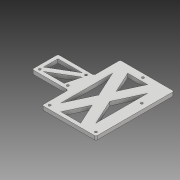
# Autodesk Inventor part: soporte_nuc_up
Saved by Autodesk Inventor 2018 (Build 220112000, 112)
## iProperties
Created: 2019-01-10
Part Number: soporte_nuc_up
Material: Genérico
Document SubType Name: Modeling
Designer: becar
Density: 1 g/cm^3
Appearance: Valor por defecto
Author: becar
Autodesk Inventor part; units mm, degrees
ref_plane "YZ Plane" through (0, 0, 0) normal (1, 0, 0) x (0, 1, 0)
ref_plane "XZ Plane" through (0, 0, 0) normal (0, 1, 0) x (-1, 0, 0)
ref_plane "XY Plane" through (0, 0, 0) normal (0, 0, 1) x (1, 0, 0)
sketch "Boceto1" plane through (0, 0, 0) normal (0, 0, 1) x (1, 0, 0)
  circle A0 centre (0, 0) radius 1.5
  line L0 (0, 0) -> (28.5, 0)
  line L1 (28.5, 0) -> (28.5, -30)
  circle A1 centre (28.5, -30) radius 1.5
  line L2 (28.5, -30) -> (28.5, -93)
  line L3 (28.5, -93) -> (31, -93)
  circle A2 centre (31, -93) radius 1.5
  line L4 (31, -93) -> (-30, -93)
  circle A3 centre (-30, -93) radius 1.5
  line L5 (-30, -98) -> (31, -98)
  line L6 (31, -98) -> (36, -98)
  line L7 (36, -98) -> (36, 0)
  line L8 (36, 0) -> (36, 5)
  line L9 (36, 5) -> (-30, 5)
  line L10 (-30, 5) -> (-35, 5)
  line L11 (-35, 5) -> (-35, -98)
  line L12 (-35, -98) -> (-30, -98)
  line L13 (-40.5, -46.5) -> (-40.5, -34.5)
  line L14 (-40.5, -46.5) -> (-40.5, -58.5)
  circle A4 centre (-40.5, -34.5) radius 1.5
  circle A5 centre (-40.5, -58.5) radius 1.5
  line L15 (-40.5, -58.5) -> (-77.5, -58.5)
  circle A6 centre (-77.5, -58.5) radius 1.5
  line L16 (-82.5, -58.5) -> (-82.5, -63.5)
  line L17 (-82.5, -63.5) -> (-35, -63.5)
  line L18 (-82.5, -58.5) -> (-82.5, -34.5)
  line L19 (-82.5, -34.5) -> (-82.5, -29.5)
  line L20 (-82.5, -29.5) -> (-38, -29.5)
  line L21 (-38, -29.5) -> (-35, -29.5)
  line L22 (-60.25, -58.5) -> (-77.5, -58.5)
  dimension "d0" = 3
  dimension "d1" = 28.5
  dimension "d2" = 30
  dimension "d3" = 3
  dimension "d4" = 63
  dimension "d5" = 2.5
  dimension "d6" = 3
  dimension "d7" = 61
  dimension "d8" = 3
  dimension "d9" = 5
  dimension "d10" = 5
  dimension "d11" = 5
  dimension "d12" = 5
  dimension "d15" = 12
  dimension "d16" = 12
  dimension "d17" = 3
  dimension "d18" = 3
  dimension "d19" = 37
  dimension "d20" = 3
  dimension "d21" = 5
  dimension "d22" = 5
  dimension "d23" = 5
  constraints: 46 end point, 9 point on line, 7 centre point, 7 coincident, 7 perpendicular, 3 horizontal, 2 collinear, 1 parallel, 1 vertical
  measures "d0" diameter of A0
  measures "d1" distance of L0.start L0.end
  measures "d2" distance of L0.end L1.end
  measures "d3" diameter of A1
  measures "d4" distance of L2.start L2.end
  measures "d5" distance of L2.end L3.end
  measures "d6" diameter of A2
  measures "d7" distance of L4.start L4.end
  measures "d8" diameter of A3
  measures "d9" distance of A3.centre L5.start
  measures "d10" distance of L5.end L6.end
  measures "d11" distance of L7.end L8.end
  measures "d12" distance of L9.end L10.end
  measures "d15" distance of L13.start L13.end
  measures "d16" distance of L13.start L14.end
  measures "d17" diameter of A4
  measures "d18" diameter of A5
  measures "d19" distance of L15.start L15.end
  measures "d20" diameter of A6
  measures "d21" distance of L22.end L16.start
  measures "d22" distance of L16.start L16.end
  measures "d23" distance of L18.end L19.end
extrude "Extrusión1" add sketch "Boceto1" along normal blind 5
sketch "Boceto2" plane through (0, 0, 0) normal (0, 0, -1) x (-1, 0, 0)
  circle A0 centre (0, 0) radius 1.5 projected
  circle A1 centre (0, 0) radius 3
  circle A2 centre (-28.5, -30) radius 1.5 projected
  circle A3 centre (-28.5, -30) radius 3
  circle A4 centre (-31, -93) radius 1.5 projected
  circle A5 centre (-31, -93) radius 3
  circle A6 centre (30, -93) radius 1.5 projected
  circle A7 centre (30, -93) radius 3
  circle A8 centre (40.5, -58.5) radius 1.5 projected
  circle A9 centre (40.5, -58.5) radius 3
  circle A10 centre (77.5, -58.5) radius 1.5 projected
  circle A11 centre (77.5, -58.5) radius 3
  circle A12 centre (40.5, -34.5) radius 1.5 projected
  circle A13 centre (40.5, -34.5) radius 3
  dimension "d28" = 6
  dimension "d29" = 6
  dimension "d30" = 6
  dimension "d31" = 6
  dimension "d32" = 6
  dimension "d33" = 6
  constraints: 7 centre point, 7 coincident
  measures "d28" diameter of A1
  measures "d29" diameter of A3
  measures "d30" diameter of A5
  measures "d31" diameter of A7
  measures "d32" diameter of A9
  measures "d33" diameter of A11
extrude "Extrusión2" cut sketch "Boceto2" against normal blind 3
sketch "Boceto3" plane through (0, 0, 0) normal (0, 0, -1) x (-1, 0, 0)
  circle A0 centre (-28.5, -30) radius 1.5 projected
  line L0 (-28.5, -30) -> (-21, -30)
  circle A1 centre (0, 0) radius 1.5 projected
  line L1 (0, 0) -> (0, -5)
  circle A2 centre (30, -93) radius 1.5 projected
  line L2 (30, -93) -> (25, -93)
  circle A3 centre (-31, -93) radius 1.5 projected
  line L3 (-31, -93) -> (-24.75, -93)
  line L4 (-24.75, -93) -> (-21, -93)
  circle A4 centre (40.5, -34.5) radius 1.5 projected
  line L5 (40.5, -34.5) -> (40.5, -39.5)
  line L6 (40.5, -34.5) -> (45.5, -34.5)
  circle A5 centre (40.5, -58.5) radius 3 projected
  line L7 (40.5, -58.5) -> (45.5, -58.5)
  circle A6 centre (77.5, -58.5) radius 1.5 projected
  line L8 (77.5, -58.5) -> (77.5, -53.5)
  line L9 (77.5, -53.5) -> (45.5, -34.5)
  line L10 (45.5, -34.5) -> (77.5, -34.5)
  line L11 (77.5, -34.5) -> (77.5, -53.5)
  line L12 (77.5, -58.5) -> (72.5, -58.5)
  line L13 (72.5, -58.5) -> (45.5, -58.5)
  line L14 (40.5, -39.5) -> (72.5, -58.5)
  line L15 (45.5, -58.5) -> (40.5, -39.5)
  line L16 (45.5, -58.5) -> (72.5, -58.5)
  line L17 (59, -58.5) -> (43, -49)
  line L18 (25, -49) -> (2, -5)
  line L19 (-21, -5) -> (-9.5, -27)
  line L20 (13.5, -49) -> (2, -27)
  line L21 (-10.5, -5) -> (2, -27)
  line L22 (-9.5, -49) -> (-21, -27)
  line L23 (25, -27) -> (12.5, -5)
  line L24 (12.5, -5) -> (25, -5)
  line L25 (25, -27) -> (25, -5)
  line L26 (13.5, -49) -> (25, -49)
  line L27 (-21, -27) -> (-9.5, -49)
  line L28 (-21, -27) -> (-21, -5)
  line L29 (-21, -93) -> (-21, -71)
  line L30 (13.5, -93) -> (-9.5, -49)
  line L31 (25, -71) -> (13.5, -49)
  line L32 (-21, -71.6828) -> (-21, -93)
  line L33 (-21, -71.6828) -> (-9.5, -93)
  line L34 (-9.5, -93) -> (-21, -93)
  line L35 (-21, -49) -> (-9.5, -49)
  line L36 (-9.5, -49) -> (13.5, -93)
  line L37 (13.5, -93) -> (2, -93)
  line L38 (25, -71) -> (25, -93)
  line L39 (2, -49) -> (25, -93)
  line L40 (-9.5, -27) -> (2, -49)
  line L41 (2, -49) -> (-9.5, -49)
  line L42 (-21, -27) -> (-21, -5)
  line L43 (-21, -49) -> (-9.5, -49)
  line L44 (-21, -49) -> (2, -93)
  line L45 (2, -93) -> (13.5, -93)
  line L46 (-9.5, -49) -> (13.5, -93)
  line L47 (2, -5) -> (0, -5)
  line L48 (-10.5, -5) -> (0, -5)
  line L49 (2, -49) -> (13.5, -49)
  line L50 (12.5, -5) -> (25, -27)
  line L51 (25, -27) -> (25, -5)
  line L52 (25, -5) -> (12.5, -5)
  line L53 (-21, -27) -> (-21, -5)
  line L54 (-21, -27) -> (-21, -5)
  line L55 (-21, -5) -> (2, -49)
  line L56 (2, -49) -> (-9.5, -49)
  line L57 (-9.5, -49) -> (-21, -27)
  dimension "d36" = 7.5
  dimension "d37" = 5
  dimension "d38" = 5
  dimension "d39" = 5
  dimension "d40" = 5
  dimension "d41" = 5
  dimension "d42" = 5
  constraints: 116 end point, 11 collinear, 6 horizontal, 5 point on line, 5 vertical, 2 midpoint, 2 parallel, 2 perpendicular
  measures "d36" distance of L0.start L0.end
  measures "d37" distance of L1.start L1.end
  measures "d38" distance of L2.start L2.end
  measures "d39" distance of L5.start L5.end
  measures "d40" distance of L5.start L6.end
  measures "d41" distance of L8.start L8.end
  measures "d42" distance of L8.start L12.end
extrude "Extrusión3" cut sketch "Boceto3" against normal blind 5 contours L10 L11 L9 | L14 L13 L17 L15 | L17 L13 L15 | L26 L20 L21 L48 L47 L18 | L30 L37 L44 L35 | L41 L22 L28 L19 L40 | L31 L38 L39 L49 | L23 L24 L25 | L29 L33 L34
fillet "Empalme1" radius 2 6 edges at (36, -98, 2.5) (-35, -98, 2.5) (-82.5, -63.5, 2.5) (-82.5, -29.5, 2.5) (-35, 5, 2.5) (36, 5, 2.5)
fillet "Empalme2" radius 2 2 edges at (-35, -63.5, 2.5) (-35, -29.5, 2.5)
sketch "Boceto4" plane through (0, 0, 0) normal (0, 0, -1) x (-1, 0, 0)
  line L0 (2, -49) -> (-21, -5) projected
  line L1 (12.5, -5) -> (25, -5) projected
  line L2 (-21, -5) -> (25, -5)
  line L3 (25, -93) -> (2, -49) projected
  line L4 (25, -5) -> (25, -93)
  line L5 (25, -93) -> (-21, -93)
  line L6 (-21, -93) -> (-21, -5)
  point P0 (0, 0)
  constraints: 8 end point, 3 perpendicular, 1 horizontal
extrude "Extrusión4" cut sketch "Boceto4" against normal blind 5
sketch "Boceto5" plane through (0, 0, 0) normal (0, 0, -1) x (-1, 0, 0)
  line L0 (-21, -5) -> (-21, -15)
  line L1 (-21, -5) -> (-11, -5)
  line L2 (25, -93) -> (15, -93)
  line L3 (15, -93) -> (-21, -15)
  line L4 (25, -93) -> (25, -83)
  line L5 (25, -83) -> (-11, -5)
  line L6 (-21, -93) -> (-21, -83)
  line L7 (-21, -93) -> (-11, -93)
  line L8 (25, -5) -> (15, -5)
  line L9 (25, -5) -> (25, -15)
  line L10 (25, -15) -> (-11, -93)
  line L11 (15, -5) -> (-21, -83)
  point P0 (0, 0)
  dimension "d49" = 10
  dimension "d50" = 10
  dimension "d51" = 10
  dimension "d52" = 10
  dimension "d53" = 10
  dimension "d54" = 10
  dimension "d55" = 10
  dimension "d56" = 10
  constraints: 24 end point, 1 parallel, 1 point on line
  measures "d49" distance of L0.start L0.end
  measures "d50" distance of L0.start L1.end
  measures "d51" distance of L2.start L2.end
  measures "d52" distance of L2.start L4.end
  measures "d53" distance of L6.start L6.end
  measures "d54" distance of L6.start L7.end
  measures "d55" distance of L8.start L8.end
  measures "d56" distance of L8.start L9.end
extrude "Extrusión5" add sketch "Boceto5" against normal blind 5
